Autodesk Fusion 360 part; units mm, degrees
(part 2 of 2)
sketch "Sketch3" plane through (0, 0, 4.8) normal (0, 0, 1) x (-1, 0, 0)
  arc A0 (-11.276, 39.5306) -> (-14.1738, 40.307) centre (-12.7249, 39.9188) ccw
  line L0 (-11.276, 39.5306) -> (-10.9973, 39.0479)
  arc A1 (-11.7738, 36.1501) -> (-10.9973, 39.0479) centre (-11.3855, 37.599) ccw
  line L1 (-11.7738, 36.1501) -> (-25.42, 28.2714)
  arc A2 (-28.3178, 29.0479) -> (-25.42, 28.2714) centre (-26.8689, 28.6596) ccw
  line L2 (-28.3178, 29.0479) -> (-28.5965, 29.5306)
  arc A3 (-27.82, 32.4283) -> (-28.5965, 29.5306) centre (-28.2083, 30.9795) ccw
  line L3 (-27.82, 32.4283) -> (-14.1738, 40.307)
  circle A4 centre (-123.5112, -37.2289) radius 1.5
  circle A5 centre (-28.2185, 125.8758) radius 1.5
  circle A6 centre (-94.9024, 87.3758) radius 1.5
  arc A7 (-10.9973, -39.0479) -> (-11.7738, -36.1501) centre (-11.3855, -37.599) ccw
  line L4 (-10.9973, -39.0479) -> (-11.276, -39.5306)
  arc A8 (-14.1738, -40.307) -> (-11.276, -39.5306) centre (-12.7249, -39.9188) ccw
  line L5 (-14.1738, -40.307) -> (-27.82, -32.4283)
  arc A9 (-28.5965, -29.5306) -> (-27.82, -32.4283) centre (-28.2083, -30.9795) ccw
  line L6 (-28.5965, -29.5306) -> (-28.3178, -29.0479)
  arc A10 (-25.42, -28.2714) -> (-28.3178, -29.0479) centre (-26.8689, -28.6596) ccw
  line L7 (-25.42, -28.2714) -> (-11.7738, -36.1501)
  circle A11 centre (123.1209, -38.5) radius 1.5
  arc A12 (-55.22, 79.8865) -> (-55.9965, 76.9888) centre (-55.6083, 78.4376) ccw
  line L8 (-55.22, 79.8865) -> (-41.5738, 87.7652)
  arc A13 (-38.676, 86.9888) -> (-41.5738, 87.7652) centre (-40.1249, 87.377) ccw
  line L9 (-38.676, 86.9888) -> (-38.3973, 86.5061)
  arc A14 (-39.1738, 83.6083) -> (-38.3973, 86.5061) centre (-38.7855, 85.0572) ccw
  line L10 (-39.1738, 83.6083) -> (-52.82, 75.7296)
  arc A15 (-55.7178, 76.5061) -> (-52.82, 75.7296) centre (-54.2689, 76.1178) ccw
  line L11 (-55.7178, 76.5061) -> (-55.9965, 76.9888)
  arc A16 (94.6725, -10) -> (96.7938, -7.8787) centre (95.7331, -8.9393) ccw
  line L12 (94.6725, -10) -> (94.1151, -10)
  arc A17 (91.9938, -7.8787) -> (94.1151, -10) centre (93.0544, -8.9393) ccw
  line L13 (91.9938, -7.8787) -> (91.9938, 7.8787)
  arc A18 (94.1151, 10) -> (91.9938, 7.8787) centre (93.0544, 8.9393) ccw
  line L14 (94.1151, 10) -> (94.6725, 10)
  arc A19 (96.7938, 7.8787) -> (94.6725, 10) centre (95.7331, 8.9393) ccw
  line L15 (96.7938, 7.8787) -> (96.7938, -7.8787)
  circle A20 centre (-28.2185, -125.8758) radius 1.5
  circle A21 centre (-94.9024, -87.3758) radius 1.5
  arc A22 (39.8725, -10) -> (41.9938, -7.8787) centre (40.9331, -8.9393) ccw
  line L16 (39.8725, -10) -> (39.3151, -10)
  arc A23 (37.1938, -7.8787) -> (39.3151, -10) centre (38.2544, -8.9393) ccw
  line L17 (37.1938, -7.8787) -> (37.1938, 7.8787)
  arc A24 (39.3151, 10) -> (37.1938, 7.8787) centre (38.2544, 8.9393) ccw
  line L18 (39.3151, 10) -> (39.8725, 10)
  arc A25 (41.9938, 7.8787) -> (39.8725, 10) centre (40.9331, 8.9393) ccw
  line L19 (41.9938, 7.8787) -> (41.9938, -7.8787)
  circle A26 centre (64.5, -111.7173) radius 1.5
  circle A27 centre (64.5, 111.7173) radius 1.5
  circle A28 centre (-123.5112, 37.2289) radius 1.5
  circle A29 centre (123.1209, 38.5) radius 1.5
  arc A30 (-52.82, -75.7296) -> (-55.7178, -76.5061) centre (-54.2689, -76.1178) ccw
  line L20 (-52.82, -75.7296) -> (-39.1738, -83.6083)
  arc A31 (-38.3973, -86.5061) -> (-39.1738, -83.6083) centre (-38.7855, -85.0572) ccw
  line L21 (-38.3973, -86.5061) -> (-38.676, -86.9888)
  arc A32 (-41.5738, -87.7652) -> (-38.676, -86.9888) centre (-40.1249, -87.377) ccw
  line L22 (-41.5738, -87.7652) -> (-55.22, -79.8865)
  arc A33 (-55.9965, -76.9888) -> (-55.22, -79.8865) centre (-55.6083, -78.4376) ccw
  line L23 (-55.9965, -76.9888) -> (-55.7178, -76.5061)
  line L24 (-42.1213, -25.5) -> (-109.5263, -25.5)
  arc A34 (-109.5263, -25.5) -> (-110.7763, -25.8349) centre (-109.5263, -28) ccw
  line L25 (-110.7763, -25.8349) -> (-125.9451, -34.5927)
  arc A35 (-125.9451, -34.5927) -> (-127.0931, -37.4646) centre (-124.6951, -36.7577) ccw
  arc A36 (-127.0931, -37.4646) -> (-96.5343, -90.76) centre (0, 0) ccw
  arc A37 (-96.5343, -90.76) -> (-92.5478, -90.2976) centre (-94.7129, -89.0476) ccw
  line L26 (-92.5478, -90.2976) -> (-83.2684, -74.2252)
  arc A38 (-80.3707, -73.4487) -> (-83.2684, -74.2252) centre (-81.8196, -73.8369) ccw
  line L27 (-80.3707, -73.4487) -> (-23.4231, -106.3274)
  arc A39 (-22.6467, -109.2252) -> (-23.4231, -106.3274) centre (-23.0349, -107.7763) ccw
  line L28 (-22.6467, -109.2252) -> (-31.9261, -125.2976)
  arc A40 (-31.9261, -125.2976) -> (-30.3333, -128.9812) centre (-29.761, -126.5476) ccw
  arc A41 (-30.3333, -128.9812) -> (126.8676, -38.2212) centre (0, 0) ccw
  arc A42 (126.8676, -38.2212) -> (124.4739, -35) centre (124.4739, -37.5) ccw
  line L29 (124.4739, -35) -> (105.9151, -35)
  arc A43 (103.7938, -32.8787) -> (105.9151, -35) centre (104.8544, -33.9393) ccw
  line L30 (103.7938, -32.8787) -> (103.7938, 32.8787)
  arc A44 (105.9151, 35) -> (103.7938, 32.8787) centre (104.8544, 33.9393) ccw
  line L31 (105.9151, 35) -> (124.4739, 35)
  arc A45 (124.4739, 35) -> (126.8676, 38.2212) centre (124.4739, 37.5) ccw
  arc A46 (126.8676, 38.2212) -> (-30.3333, 128.9812) centre (0, 0) ccw
  arc A47 (-30.3333, 128.9812) -> (-31.9261, 125.2976) centre (-29.761, 126.5476) ccw
  line L32 (-31.9261, 125.2976) -> (-22.6467, 109.2252)
  arc A48 (-23.4231, 106.3274) -> (-22.6467, 109.2252) centre (-23.0349, 107.7763) ccw
  line L33 (-23.4231, 106.3274) -> (-80.3707, 73.4487)
  arc A49 (-83.2684, 74.2252) -> (-80.3707, 73.4487) centre (-81.8196, 73.8369) ccw
  line L34 (-83.2684, 74.2252) -> (-92.5478, 90.2976)
  arc A50 (-92.5478, 90.2976) -> (-96.5343, 90.76) centre (-94.7129, 89.0476) ccw
  arc A51 (-96.5343, 90.76) -> (-127.0931, 37.4646) centre (0, 0) ccw
  arc A52 (-127.0931, 37.4646) -> (-125.9451, 34.5927) centre (-124.6951, 36.7577) ccw
  line L35 (-125.9451, 34.5927) -> (-110.7763, 25.8349)
  arc A53 (-110.7763, 25.8349) -> (-109.5263, 25.5) centre (-109.5263, 28) ccw
  line L36 (-109.5263, 25.5) -> (-42.1213, 25.5)
  arc A54 (-40, 23.3787) -> (-42.1213, 25.5) centre (-41.0607, 24.4393) ccw
  line L37 (-40, 23.3787) -> (-40, 20.8)
  arc A55 (-40, 20.8) -> (-37.5, 18.3) centre (-37.5, 20.8) ccw
  line L38 (-37.5, 18.3) -> (-34.1213, 18.3)
  arc A56 (-32, 16.1787) -> (-34.1213, 18.3) centre (-33.0607, 17.2393) ccw
  line L39 (-32, 16.1787) -> (-32, -16.1787)
  arc A57 (-34.1213, -18.3) -> (-32, -16.1787) centre (-33.0607, -17.2393) ccw
  line L40 (-34.1213, -18.3) -> (-37.5, -18.3)
  arc A58 (-37.5, -18.3) -> (-40, -20.8) centre (-37.5, -20.8) ccw
  line L41 (-40, -20.8) -> (-40, -23.3787)
  arc A59 (-42.1213, -25.5) -> (-40, -23.3787) centre (-41.0607, -24.4393) ccw
  line L42 (103.7938, 35) -> (103.7938, -35)
  line L43 (0, 0) -> (132.5, 0)
  line L44 (91.7938, -20) -> (19.1938, -20) construction
  line L45 (19.1938, -20) -> (19.1938, 20) construction
  line L46 (19.1938, 20) -> (91.7938, 20) construction
  line L47 (91.7938, 20) -> (91.7938, -20) construction
  line L48 (127.7938, -35) -> (127.7938, 35) construction
  line L49 (91.7938, -20) -> (19.1938, 20) construction
  line L50 (82.5688, 22) -> (21.1938, 22) construction
  line L51 (21.1938, 22) -> (21.1938, 51.625) construction
  line L52 (21.1938, 51.625) -> (82.5688, 51.625) construction
  line L53 (82.5688, 51.625) -> (82.5688, 22) construction
  circle A60 centre (50.5438, 24.337) radius 1.1
  circle A61 centre (68.4688, 49.121) radius 1.1
  circle A62 centre (41.2968, 49.4) radius 1.1
  point P0 (55.4938, 0)
  dimension "d151" = 72.6
  dimension "d152" = 40
  dimension "d153" = 108.6
  dimension "d154" = 61.375
  dimension "d155" = 29.625
  dimension "d156" = 2
  dimension "d158" = 2
  dimension "d159" = 2.2
  dimension "d160" = 2.2
  dimension "d161" = 2.2
  dimension "d162" = 2.337
  dimension "d163" = 2.504
  dimension "d164" = 2.225
  dimension "d165" = 29.35
  dimension "d166" = 20.103
  dimension "d167" = 14.1
  constraint horizontal L44
  constraint vertical L45
  constraint horizontal L46
  constraint vertical L47
  constraint midpoint L49 P0
  constraint coincident L43 P0
  constraint horizontal L50
  constraint vertical L51
  constraint horizontal L52
  constraint vertical L53
  measures "d151" distance of L44.start L44.end
  measures "d152" distance of L44.start L46.end
  measures "d153" distance of L45 L48
  measures "d154" distance of L50.start L50.end
  measures "d155" distance of L50.start L52.end
  measures "d156" distance of L46 L50
  measures "d158" distance of L45 L51
  measures "d159" diameter of A60
  measures "d160" diameter of A61
  measures "d161" diameter of A62
  measures "d162" distance of L50 A60.centre
  measures "d163" distance of L52 A61.centre
  measures "d164" distance of L52 A62.centre
  measures "d165" distance of L51 A60.centre
  measures "d166" distance of L51 A62.centre
  measures "d167" distance of L53 A61.centre
extrude "Extrude3" cut sketch "Sketch3" against normal through all contours A60 | A61 | A62
sketch "Sketch4" plane through (0, 0, 4.8) normal (0, 0, 1) x (-1, 0, 0)
  circle A0 centre (41.2968, 49.4) radius 1.1
  circle A1 centre (68.4688, 49.121) radius 1.1
  circle A2 centre (50.5438, 24.337) radius 1.1
  arc A3 (-11.276, 39.5306) -> (-14.1738, 40.307) centre (-12.7249, 39.9188) ccw
  line L0 (-11.276, 39.5306) -> (-10.9973, 39.0479)
  arc A4 (-11.7738, 36.1501) -> (-10.9973, 39.0479) centre (-11.3855, 37.599) ccw
  line L1 (-11.7738, 36.1501) -> (-25.42, 28.2714)
  arc A5 (-28.3178, 29.0479) -> (-25.42, 28.2714) centre (-26.8689, 28.6596) ccw
  line L2 (-28.3178, 29.0479) -> (-28.5965, 29.5306)
  arc A6 (-27.82, 32.4283) -> (-28.5965, 29.5306) centre (-28.2083, 30.9795) ccw
  line L3 (-27.82, 32.4283) -> (-14.1738, 40.307)
  circle A7 centre (-123.5112, -37.2289) radius 1.5
  circle A8 centre (-28.2185, 125.8758) radius 1.5
  circle A9 centre (-94.9024, 87.3758) radius 1.5
  arc A10 (-10.9973, -39.0479) -> (-11.7738, -36.1501) centre (-11.3855, -37.599) ccw
  line L4 (-10.9973, -39.0479) -> (-11.276, -39.5306)
  arc A11 (-14.1738, -40.307) -> (-11.276, -39.5306) centre (-12.7249, -39.9188) ccw
  line L5 (-14.1738, -40.307) -> (-27.82, -32.4283)
  arc A12 (-28.5965, -29.5306) -> (-27.82, -32.4283) centre (-28.2083, -30.9795) ccw
  line L6 (-28.5965, -29.5306) -> (-28.3178, -29.0479)
  arc A13 (-25.42, -28.2714) -> (-28.3178, -29.0479) centre (-26.8689, -28.6596) ccw
  line L7 (-25.42, -28.2714) -> (-11.7738, -36.1501)
  circle A14 centre (123.1209, -38.5) radius 1.5
  arc A15 (-55.22, 79.8865) -> (-55.9965, 76.9888) centre (-55.6083, 78.4376) ccw
  line L8 (-55.22, 79.8865) -> (-41.5738, 87.7652)
  arc A16 (-38.676, 86.9888) -> (-41.5738, 87.7652) centre (-40.1249, 87.377) ccw
  line L9 (-38.676, 86.9888) -> (-38.3973, 86.5061)
  arc A17 (-39.1738, 83.6083) -> (-38.3973, 86.5061) centre (-38.7855, 85.0572) ccw
  line L10 (-39.1738, 83.6083) -> (-52.82, 75.7296)
  arc A18 (-55.7178, 76.5061) -> (-52.82, 75.7296) centre (-54.2689, 76.1178) ccw
  line L11 (-55.7178, 76.5061) -> (-55.9965, 76.9888)
  arc A19 (94.6725, -10) -> (96.7938, -7.8787) centre (95.7331, -8.9393) ccw
  line L12 (94.6725, -10) -> (94.1151, -10)
  arc A20 (91.9938, -7.8787) -> (94.1151, -10) centre (93.0544, -8.9393) ccw
  line L13 (91.9938, -7.8787) -> (91.9938, 7.8787)
  arc A21 (94.1151, 10) -> (91.9938, 7.8787) centre (93.0544, 8.9393) ccw
  line L14 (94.1151, 10) -> (94.6725, 10)
  arc A22 (96.7938, 7.8787) -> (94.6725, 10) centre (95.7331, 8.9393) ccw
  line L15 (96.7938, 7.8787) -> (96.7938, -7.8787)
  circle A23 centre (-28.2185, -125.8758) radius 1.5
  circle A24 centre (-94.9024, -87.3758) radius 1.5
  arc A25 (39.8725, -10) -> (41.9938, -7.8787) centre (40.9331, -8.9393) ccw
  line L16 (39.8725, -10) -> (39.3151, -10)
  arc A26 (37.1938, -7.8787) -> (39.3151, -10) centre (38.2544, -8.9393) ccw
  line L17 (37.1938, -7.8787) -> (37.1938, 7.8787)
  arc A27 (39.3151, 10) -> (37.1938, 7.8787) centre (38.2544, 8.9393) ccw
  line L18 (39.3151, 10) -> (39.8725, 10)
  arc A28 (41.9938, 7.8787) -> (39.8725, 10) centre (40.9331, 8.9393) ccw
  line L19 (41.9938, 7.8787) -> (41.9938, -7.8787)
  circle A29 centre (64.5, -111.7173) radius 1.5
  circle A30 centre (64.5, 111.7173) radius 1.5
  circle A31 centre (-123.5112, 37.2289) radius 1.5
  circle A32 centre (123.1209, 38.5) radius 1.5
  arc A33 (-52.82, -75.7296) -> (-55.7178, -76.5061) centre (-54.2689, -76.1178) ccw
  line L20 (-52.82, -75.7296) -> (-39.1738, -83.6083)
  arc A34 (-38.3973, -86.5061) -> (-39.1738, -83.6083) centre (-38.7855, -85.0572) ccw
  line L21 (-38.3973, -86.5061) -> (-38.676, -86.9888)
  arc A35 (-41.5738, -87.7652) -> (-38.676, -86.9888) centre (-40.1249, -87.377) ccw
  line L22 (-41.5738, -87.7652) -> (-55.22, -79.8865)
  arc A36 (-55.9965, -76.9888) -> (-55.22, -79.8865) centre (-55.6083, -78.4376) ccw
  line L23 (-55.9965, -76.9888) -> (-55.7178, -76.5061)
  line L24 (-42.1213, -25.5) -> (-109.5263, -25.5)
  arc A37 (-109.5263, -25.5) -> (-110.7763, -25.8349) centre (-109.5263, -28) ccw
  line L25 (-110.7763, -25.8349) -> (-125.9451, -34.5927)
  arc A38 (-125.9451, -34.5927) -> (-127.0931, -37.4646) centre (-124.6951, -36.7577) ccw
  arc A39 (-127.0931, -37.4646) -> (-96.5343, -90.76) centre (0, 0) ccw
  arc A40 (-96.5343, -90.76) -> (-92.5478, -90.2976) centre (-94.7129, -89.0476) ccw
  line L26 (-92.5478, -90.2976) -> (-83.2684, -74.2252)
  arc A41 (-80.3707, -73.4487) -> (-83.2684, -74.2252) centre (-81.8196, -73.8369) ccw
  line L27 (-80.3707, -73.4487) -> (-23.4231, -106.3274)
  arc A42 (-22.6467, -109.2252) -> (-23.4231, -106.3274) centre (-23.0349, -107.7763) ccw
  line L28 (-22.6467, -109.2252) -> (-31.9261, -125.2976)
  arc A43 (-31.9261, -125.2976) -> (-30.3333, -128.9812) centre (-29.761, -126.5476) ccw
  arc A44 (-30.3333, -128.9812) -> (126.8676, -38.2212) centre (0, 0) ccw
  arc A45 (126.8676, -38.2212) -> (124.4739, -35) centre (124.4739, -37.5) ccw
  line L29 (124.4739, -35) -> (105.9151, -35)
  arc A46 (103.7938, -32.8787) -> (105.9151, -35) centre (104.8544, -33.9393) ccw
  line L30 (103.7938, -32.8787) -> (103.7938, 32.8787)
  arc A47 (105.9151, 35) -> (103.7938, 32.8787) centre (104.8544, 33.9393) ccw
  line L31 (105.9151, 35) -> (124.4739, 35)
  arc A48 (124.4739, 35) -> (126.8676, 38.2212) centre (124.4739, 37.5) ccw
  arc A49 (126.8676, 38.2212) -> (-30.3333, 128.9812) centre (0, 0) ccw
  arc A50 (-30.3333, 128.9812) -> (-31.9261, 125.2976) centre (-29.761, 126.5476) ccw
  line L32 (-31.9261, 125.2976) -> (-22.6467, 109.2252)
  arc A51 (-23.4231, 106.3274) -> (-22.6467, 109.2252) centre (-23.0349, 107.7763) ccw
  line L33 (-23.4231, 106.3274) -> (-80.3707, 73.4487)
  arc A52 (-83.2684, 74.2252) -> (-80.3707, 73.4487) centre (-81.8196, 73.8369) ccw
  line L34 (-83.2684, 74.2252) -> (-92.5478, 90.2976)
  arc A53 (-92.5478, 90.2976) -> (-96.5343, 90.76) centre (-94.7129, 89.0476) ccw
  arc A54 (-96.5343, 90.76) -> (-127.0931, 37.4646) centre (0, 0) ccw
  arc A55 (-127.0931, 37.4646) -> (-125.9451, 34.5927) centre (-124.6951, 36.7577) ccw
  line L35 (-125.9451, 34.5927) -> (-110.7763, 25.8349)
  arc A56 (-110.7763, 25.8349) -> (-109.5263, 25.5) centre (-109.5263, 28) ccw
  line L36 (-109.5263, 25.5) -> (-42.1213, 25.5)
  arc A57 (-40, 23.3787) -> (-42.1213, 25.5) centre (-41.0607, 24.4393) ccw
  line L37 (-40, 23.3787) -> (-40, 20.8)
  arc A58 (-40, 20.8) -> (-37.5, 18.3) centre (-37.5, 20.8) ccw
  line L38 (-37.5, 18.3) -> (-34.1213, 18.3)
  arc A59 (-32, 16.1787) -> (-34.1213, 18.3) centre (-33.0607, 17.2393) ccw
  line L39 (-32, 16.1787) -> (-32, -16.1787)
  arc A60 (-34.1213, -18.3) -> (-32, -16.1787) centre (-33.0607, -17.2393) ccw
  line L40 (-34.1213, -18.3) -> (-37.5, -18.3)
  arc A61 (-37.5, -18.3) -> (-40, -20.8) centre (-37.5, -20.8) ccw
  line L41 (-40, -20.8) -> (-40, -23.3787)
  arc A62 (-42.1213, -25.5) -> (-40, -23.3787) centre (-41.0607, -24.4393) ccw
  circle A63 centre (-100, 31.3) radius 1.5
  line L42 (-105, -25.5) -> (-105, 25.5)
  line L43 (-130.0231, 25.5) -> (-40, 25.5)
  circle A64 centre (-100, -31.3) radius 1.5
  line L44 (-42.1213, -25.5) -> (-109.5263, -25.5)
  dimension "d169" = 3
  dimension "d170" = 5
  dimension "d171" = 5.8
  dimension "d172" = 3
  dimension "d173" = 5
  dimension "d174" = 5.8
  measures "d169" diameter of A63
  measures "d170" distance of A63.centre L42
  measures "d171" distance of A63.centre L43
  measures "d172" diameter of A64
  measures "d173" horizontal distance of L42.start A64.centre
  measures "d174" distance of A64.centre L44
extrude "Extrude4" cut sketch "Sketch4" against normal through all contours A63 | A64
